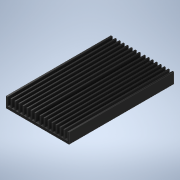
# Autodesk Inventor part: heatsink
Saved by Autodesk Inventor 2020 (Build 240168000, 168)
## iProperties
Created: 2020-11-25
Part Number: heatsink
Material: Aluminum 6061
Document SubType Name: Modeling
Designer: Curtis
Density: 2.7 g/cm^3
Appearance: Aluminum - Flat
Author: Curtis
Autodesk Inventor part; units mm, degrees
ref_plane "YZ Plane" through (0, 0, 0) normal (1, 0, 0) x (0, 1, 0)
ref_plane "XZ Plane" through (0, 0, 0) normal (0, 1, 0) x (-1, 0, 0)
ref_plane "XY Plane" through (0, 0, 0) normal (0, 0, 1) x (1, 0, 0)
sketch "Sketch1" plane through (0, 0, 0) normal (0, 1, 0) x (-1, 0, 0)
  line L0 (0, 0) -> (60, 0)
  line L1 (60, 0) -> (60, -100)
  line L2 (60, -100) -> (0, -100)
  line L3 (0, -100) -> (0, 0)
  dimension "d0" = 60
  dimension "d1" = 100
  constraints: 8 end point, 2 parallel, 1 horizontal, 1 perpendicular
  measures "d0" distance of L1.end L2.end
  measures "d1" distance of L0.end L1.end
extrude "Extrusion1" add sketch "Sketch1" along normal blind 10
sketch "Sketch2" plane through (0, 10, 0) normal (0, 1, 0) x (1, 0, 0)
  line L0 (-60, 0) -> (0, 0) projected
  line L1 (-30, 0) -> (-30, 100)
  line L2 (0, 100) -> (-60, 100) projected
  line L3 (-31.9, 0) -> (-28.1, 0)
  line L4 (-28.1, 0) -> (-28.1, 100)
  line L5 (-28.1, 100) -> (-31.9, 100)
  line L6 (-31.9, 100) -> (-31.9, 0)
  line L7 (-31.9, 0) -> (-28.1, 100) construction
  line L8 (-28.1, 0) -> (-31.9, 100) construction
  line L9 (-32.9, 0) -> (-35.72, 0)
  line L10 (-35.72, 0) -> (-35.72, 100)
  line L11 (-35.72, 100) -> (-32.9, 100)
  line L12 (-32.9, 100) -> (-32.9, 0)
  line L13 (-32.9, 0) -> (-35.72, 100) construction
  line L14 (-35.72, 0) -> (-32.9, 100) construction
  line L15 (-39.54, 0) -> (-36.72, 0)
  line L16 (-36.72, 0) -> (-36.72, 100)
  line L17 (-36.72, 100) -> (-39.54, 100)
  line L18 (-39.54, 100) -> (-39.54, 0)
  line L19 (-39.54, 0) -> (-36.72, 100) construction
  line L20 (-36.72, 0) -> (-39.54, 100) construction
  line L21 (-43.36, 0) -> (-40.54, 0)
  line L22 (-40.54, 0) -> (-40.54, 100)
  line L23 (-40.54, 100) -> (-43.36, 100)
  line L24 (-43.36, 100) -> (-43.36, 0)
  line L25 (-43.36, 0) -> (-40.54, 100) construction
  line L26 (-40.54, 0) -> (-43.36, 100) construction
  line L27 (-47.18, 0) -> (-44.36, 0)
  line L28 (-44.36, 0) -> (-44.36, 100)
  line L29 (-44.36, 100) -> (-47.18, 100)
  line L30 (-47.18, 100) -> (-47.18, 0)
  line L31 (-47.18, 0) -> (-44.36, 100) construction
  line L32 (-44.36, 0) -> (-47.18, 100) construction
  line L33 (-51, 0) -> (-48.18, 0)
  line L34 (-48.18, 0) -> (-48.18, 100)
  line L35 (-48.18, 100) -> (-51, 100)
  line L36 (-51, 100) -> (-51, 0)
  line L37 (-51, 0) -> (-48.18, 100) construction
  line L38 (-48.18, 0) -> (-51, 100) construction
  line L39 (-54.82, 0) -> (-52, 0)
  line L40 (-52, 0) -> (-52, 100)
  line L41 (-52, 100) -> (-54.82, 100)
  line L42 (-54.82, 100) -> (-54.82, 0)
  line L43 (-54.82, 0) -> (-52, 100) construction
  line L44 (-52, 0) -> (-54.82, 100) construction
  line L45 (-58.64, 0) -> (-55.82, 0)
  line L46 (-55.82, 0) -> (-55.82, 100)
  line L47 (-55.82, 100) -> (-58.64, 100)
  line L48 (-58.64, 100) -> (-58.64, 0)
  line L49 (-58.64, 0) -> (-55.82, 100) construction
  line L50 (-55.82, 0) -> (-58.64, 100) construction
  line L51 (-31.9, 0) -> (-31.9, 100)
  line L52 (-28.1, 100) -> (-28.1, 0)
  line L53 (-28.1, 0) -> (-31.9, 100) construction
  line L54 (-31.9, 0) -> (-28.1, 100) construction
  line L55 (-24.28, 0) -> (-24.28, 100)
  line L56 (-27.1, 100) -> (-27.1, 0)
  line L57 (-27.1, 0) -> (-24.28, 100) construction
  line L58 (-24.28, 0) -> (-27.1, 100) construction
  line L59 (-23.28, 0) -> (-23.28, 100)
  line L60 (-20.46, 100) -> (-20.46, 0)
  line L61 (-20.46, 0) -> (-23.28, 100) construction
  line L62 (-23.28, 0) -> (-20.46, 100) construction
  line L63 (-19.46, 0) -> (-19.46, 100)
  line L64 (-16.64, 100) -> (-16.64, 0)
  line L65 (-16.64, 0) -> (-19.46, 100) construction
  line L66 (-19.46, 0) -> (-16.64, 100) construction
  line L67 (-15.64, 0) -> (-15.64, 100)
  line L68 (-12.82, 100) -> (-12.82, 0)
  line L69 (-12.82, 0) -> (-15.64, 100) construction
  line L70 (-15.64, 0) -> (-12.82, 100) construction
  line L71 (-11.82, 0) -> (-11.82, 100)
  line L72 (-9, 100) -> (-9, 0)
  line L73 (-9, 0) -> (-11.82, 100) construction
  line L74 (-11.82, 0) -> (-9, 100) construction
  line L75 (-8, 0) -> (-8, 100)
  line L76 (-5.18, 100) -> (-5.18, 0)
  line L77 (-5.18, 0) -> (-8, 100) construction
  line L78 (-8, 0) -> (-5.18, 100) construction
  line L79 (-4.18, 0) -> (-4.18, 100)
  line L80 (-1.36, 100) -> (-1.36, 0)
  line L81 (-1.36, 0) -> (-4.18, 100) construction
  line L82 (-4.18, 0) -> (-1.36, 100) construction
  line L83 (-60, 100) -> (-60, 0) projected
  point P0 (-30, 50)
  point P1 (-34.31, 50)
  point P2 (-38.13, 50)
  point P3 (-41.95, 50)
  point P4 (-45.77, 50)
  point P5 (-49.59, 50)
  point P6 (-53.41, 50)
  point P7 (-57.23, 50)
  point P8 (-25.69, 50)
  point P9 (-21.87, 50)
  point P10 (-18.05, 50)
  point P11 (-14.23, 50)
  point P12 (-10.41, 50)
  point P13 (-6.59, 50)
  point P14 (-2.77, 50)
  point P15 (-1.36, 0)
  point P16 (-1.36, 100)
  point P17 (-4.18, 100)
  point P18 (-4.18, 0)
  point P19 (-5.18, 0)
  point P20 (-5.18, 100)
  point P21 (-8, 100)
  point P22 (-8, 0)
  point P23 (-9, 0)
  point P24 (-9, 100)
  point P25 (-11.82, 100)
  point P26 (-11.82, 0)
  point P27 (-12.82, 0)
  point P28 (-12.82, 100)
  point P29 (-15.64, 100)
  point P30 (-15.64, 0)
  point P31 (-16.64, 0)
  point P32 (-16.64, 100)
  point P33 (-19.46, 100)
  point P34 (-19.46, 0)
  point P35 (-23.28, 0)
  point P36 (-20.46, 0)
  point P37 (-27.1, 0)
  point P38 (-24.28, 0)
  point P39 (-31.9, 0)
  point P40 (-28.1, 0)
  point P41 (-32.9, 0)
  point P42 (-35.72, 0)
  point P43 (-39.54, 0)
  point P44 (-36.72, 0)
  point P45 (-43.36, 0)
  point P46 (-40.54, 0)
  point P47 (-47.18, 0)
  point P48 (-44.36, 0)
  point P49 (-51, 0)
  point P50 (-48.18, 0)
  point P51 (-54.82, 100)
  point P52 (-54.82, 0)
  point P53 (-52, 0)
  point P54 (-52, 100)
  point P55 (-58.64, 100)
  point P56 (-58.64, 0)
  point P57 (-55.82, 0)
  point P58 (-55.82, 100)
  dimension "d4" = 3.8
  dimension "d5" = 100
  dimension "d6" = 2.82
  dimension "d7" = 1
  dimension "d8" = 100
  dimension "d9" = 2.82
  dimension "d10" = 1
  dimension "d11" = 2.82
  dimension "d12" = 1
  dimension "d13" = 2.82
  dimension "d14" = 100
  dimension "d15" = 1
  dimension "d16" = 2.82
  dimension "d17" = 100
  dimension "d18" = 1
  dimension "d19" = 2.82
  dimension "d20" = 100
  dimension "d21" = 1
  dimension "d22" = 2.82
  dimension "d23" = 100
  dimension "d24" = 1
  dimension "d27" = 1.36
  dimension "d28" = 0
  dimension "d29" = 0
  dimension "d30" = 100
  dimension "d31" = 100
  constraints: 162 end point, 39 symmetric about line, 31 midpoint, 16 parallel, 8 horizontal, 8 perpendicular, 7 other
  measures "d4" distance of L5.end L4.end
  measures "d5" distance of L4.end L3.end
  measures "d6" distance of L10.end L11.end
  measures "d7" distance between parallel lines of L6 L12
  measures "d8" distance of L9.end L10.end
  measures "d9" distance of L17.end L16.end
  measures "d10" distance between parallel lines of L10 L16
  measures "d11" distance of L23.end L22.end
  measures "d12" distance between parallel lines of L18 L22
  measures "d13" distance of L29.end L28.end
  measures "d14" distance of L28.end L27.end
  measures "d15" distance between parallel lines of L24 L28
  measures "d16" distance of L35.end L34.end
  measures "d17" distance of L34.end L33.end
  measures "d18" distance between parallel lines of L30 L34
  measures "d19" distance of L41.end L40.end
  measures "d20" distance of L40.end L39.end
  measures "d21" distance between parallel lines of L36 L40
  measures "d22" distance of L47.end L46.end
  measures "d23" distance of L46.end L45.end
  measures "d24" distance between parallel lines of L42 L46
  measures "d27" distance between parallel lines of L48 L83
  measures "d28" vertical extent of L45
  measures "d29" vertical extent of L39
  measures "d30" distance of L21.end L22.end
  measures "d31" distance of L15.end L16.end
extrude "Extrusion2" cut sketch "Sketch2" against normal blind 7.8 contours L48 L2 L46 L0 | L42 L2 L40 L0 | L36 L2 L34 L0 | L30 L2 L28 L0 | L24 L2 L22 L0 | L18 L2 L16 L0 | L10 L2 L12 L0 | L6 L2 L1 L0 | L1 L2 L4 L0 | L56 L2 L55 L0 | L59 L2 L60 L0 | L63 L2 L64 L0 | L67 L2 L68 L0 | L71 L2 L72 L0 | L75 L2 L76 L0 | L79 L2 L80 L0
body "Solid1"
